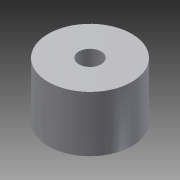
# Autodesk Inventor part: 滚子
Saved by Autodesk Inventor 2013 (Build 170138000, 138)
## iProperties
Created: 2012-09-25
Part Number: 滚子
Material: PVC 管
Document SubType Name: Modeling
Designer: Zhensheng
Density: 7.85 g/cm^3
Author: Zhensheng
Autodesk Inventor part; units mm, degrees
ref_plane "YZ Plane" through (0, 0, 0) normal (1, 0, 0) x (0, 1, 0)
ref_plane "XZ Plane" through (0, 0, 0) normal (0, 1, 0) x (-1, 0, 0)
ref_plane "XY Plane" through (0, 0, 0) normal (0, 0, 1) x (1, 0, 0)
sketch "草图1" plane through (0, 0, 0) normal (0, 0, 1) x (1, 0, 0)
  circle A0 centre (0, 0) radius 7.5
  dimension "直径" = 15
  constraints: 1 centre point, 1 coincident
  measures "直径" diameter of A0
extrude "拉伸1" add sketch "草图1" along normal mid plane 10
sketch "草图2" plane through (0, 0, 5) normal (0, 0, 1) x (1, 0, 0)
  circle A0 centre (0, 0) radius 2
  dimension "孔径" = 4
  constraints: 1 centre point, 1 coincident
  measures "孔径" diameter of A0
extrude "拉伸2" cut sketch "草图2" along normal through all both and the other way through all
